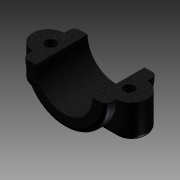
# Autodesk Inventor part: Abrazadera
Saved by Autodesk Inventor 2016 (Build 200138000, 138)
## iProperties
Created: 2013-07-10
Part Number: Abrazadera
Material: Generic
Document SubType Name: Modeling
Designer: Luis
Density: 1 g/cm^3
Appearance: Fine Textured - Black
Author: Luis
Autodesk Inventor part; units mm, degrees
ref_plane "YZ Plane" through (0, 0, 0) normal (1, 0, 0) x (0, 1, 0)
ref_plane "XZ Plane" through (0, 0, 0) normal (0, 1, 0) x (-1, 0, 0)
sketch "Sketch1" plane through (0, 0, 0) normal (0, 0, 1) x (1, 0, 0)
  arc A0 (3.8592, 10.1235) -> (3.8, 10.125) centre (3.8, 8.925) ccw construction
  line L0 (1.2, 10.125) -> (3.8, 10.125) construction
  arc A1 (1.2, 10.125) -> (0, 8.925) centre (1.2, 8.925) ccw construction
  line L1 (0, 6) -> (0, 8.925) construction
  arc A2 (0, 6) -> (0, -6) centre (0, 0) ccw
  line L2 (0, -8.925) -> (0, -6) construction
  arc A3 (0, -8.925) -> (1.2, -10.125) centre (1.2, -8.925) ccw construction
  line L3 (1.2, -10.125) -> (3.8, -10.125) construction
  arc A4 (3.8, -10.125) -> (3.8592, -10.1235) centre (3.8, -8.925) ccw construction
  line L4 (3.8592, 10.1235) -> (3.8592, -10.1235) construction
  circle A5 centre (1, 0) radius 2
  arc A6 (28.2, 10.125) -> (28.1408, 10.1235) centre (28.2, 8.925) ccw
  line L5 (28.1408, -10.1235) -> (28.1408, 10.1235)
  arc A7 (28.1408, -10.1235) -> (28.2, -10.125) centre (28.2, -8.925) ccw
  line L6 (28.2, -10.125) -> (30.8, -10.125)
  arc A8 (30.8, -10.125) -> (32, -8.925) centre (30.8, -8.925) ccw
  line L7 (32, -8.925) -> (32, -6)
  arc A9 (32, -6) -> (32, 6) centre (32, 0) ccw
  line L8 (32, 6) -> (32, 8.925)
  arc A10 (32, 8.925) -> (30.8, 10.125) centre (30.8, 8.925) ccw
  line L9 (28.2, 10.125) -> (30.8, 10.125)
  circle A11 centre (31, 0) radius 2
  line L10 (5.0533, -8.925) -> (5.0533, 8.925) construction
  line L11 (26.9467, 8.925) -> (26.9467, -8.925)
  line L12 (0, -6) -> (3.8592, -6)
  line L13 (0, 6) -> (3.8592, 6)
  line L14 (3.8592, -6) -> (3.8592, 6)
  point P0 (25.5, -25.375)
  constraints: 30 end point, 20 point on circle, 12 centre point, 2 perpendicular, 2 point on line, 2 tangent, 1 collinear
sketch "Sketch2" plane through (0, 0, 0) normal (0, 1, 0) x (-1, 0, 0)
  arc A0 (-26.9467, 0) -> (-5.0533, 0) centre (-16, 0) ccw
  arc A1 (-32, 0) -> (0, 0) centre (-16, 0) ccw
  line L0 (-28.1408, 0) -> (-26.9467, 0)
  line L1 (-5.0533, 0) -> (-3.8592, 0)
  line L2 (0, 0) -> (-5.0533, 0)
  line L3 (-26.9467, 0) -> (-32, 0)
  point P0 (-26.9467, 0)
  constraints: 8 end point, 5 point on circle, 4 collinear, 2 centre point, 1 coincident
extrude "Extrusion1" add sketch "Sketch2" along normal mid plane 20
extrude "Extrusion2" add sketch "Sketch1" against normal blind 13 contours L13 L14 L12 A2
sketch "Sketch3" plane through (3.8592, -6, -10.4211) normal (1, 0, 0) x (0, 0, -1)
  line L0 (0, 0) -> (0, 12) projected
  line L1 (0, 0) -> (2.5789, 0) projected
  line L2 (2.5789, 0) -> (2.5789, 12) projected
  line L3 (0, 12) -> (2.5789, 12) projected
  point P0 (-10.4211, 6)
extrude "Extrusion3" add sketch "Sketch3" along normal blind 5
ref_plane "Work Plane3" through (16, 10, 0) normal (-1, 0, 0) x (0, -1, 0)
ref_plane "Work Plane1" through (0, 10, 0) normal (-1, 0, 0) x (0, -1, 0)
ref_plane "Work Plane2" through (32, 10, 0) normal (-1, 0, 0) x (0, -1, 0)
mirror "Mirror1" about plane through (16, 10, 0) normal (-1, 0, 0) of "Extrusion3", "Extrusion2"
extrude "Extrusion4" cut sketch "Sketch1" against normal through all contours A5
mirror "Mirror2" about plane through (16, 10, 0) normal (-1, 0, 0) of "Extrusion4"
fillet "Fillet1" radius 2 8 edges at (3.3363, -6, -13) (3.3363, 6, -13) (-6, 0, -13) (28.6637, -6, -13) (28.6637, 6, -13) (38, 0, -13) (16, 10, -16) (16, -10, -16)
body "Solid1"
